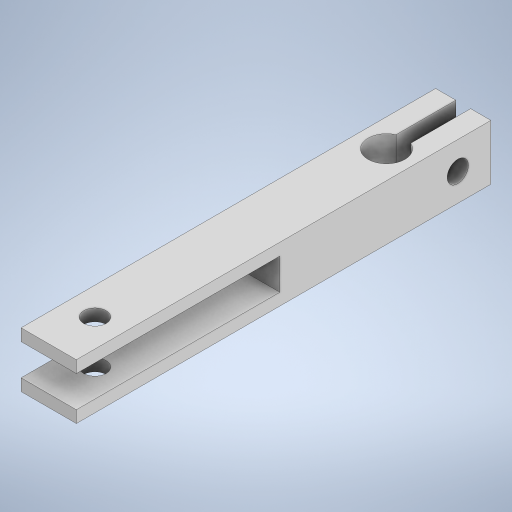
# Autodesk Inventor part: LInk1
Saved by Autodesk Inventor 2024 (Build 280153000, 153)
## iProperties
Created: 2023-12-17
Part Number: LInk1
Material: Generic
Document SubType Name: Modeling
Designer: pratikhya
Density: 1 g/cm^3
Appearance: Default
Author: pratikhya
Autodesk Inventor part; units mm, degrees
ref_plane "YZ Plane" through (0, 0, 0) normal (1, 0, 0) x (0, 1, 0)
ref_plane "XZ Plane" through (0, 0, 0) normal (0, 1, 0) x (-1, 0, 0)
ref_plane "XY Plane" through (0, 0, 0) normal (0, 0, 1) x (1, 0, 0)
sketch "Sketch1" plane through (0, 0, 0) normal (0, 1, 0) x (-1, 0, 0)
  point P0 (0, 0)
sketch "Sketch2" plane through (0, 0, 0) normal (0, 1, 0) x (-1, 0, 0)
  line L0 (2.7724, 24.8182) -> (-3.2276, 24.8182)
  line L1 (2.7724, 24.8182) -> (2.7724, -20.1818)
  line L2 (-3.2276, 24.8182) -> (-3.2276, -20.1818)
  line L3 (-3.2276, -20.1818) -> (-1.0276, -20.1818)
  line L4 (-1.0276, -20.1818) -> (-1.0276, -13.6818)
  line L5 (2.7724, -20.1818) -> (0.5724, -20.1818)
  line L6 (0.5724, -20.1818) -> (0.5724, -13.6818)
  arc A0 (0.5724, -13.6818) -> (-1.0276, -13.6818) centre (-0.2276, -11.8488) ccw
  point P0 (0, 0)
  dimension "d0" = 6
  dimension "d1" = 45
  dimension "d2" = 45
  dimension "d3" = 2.2
  dimension "d4" = 2.2
  dimension "d5" = 6.5
  dimension "d6" = 2
  constraints: 14 end point, 3 vertical, 2 horizontal, 2 perpendicular, 2 point on circle, 1 centre point
  measures "d0" distance of L0.start L0.end
  measures "d1" distance of L0.start L1.end
  measures "d2" distance of L0.end L2.end
  measures "d3" distance of L2.end L3.end
  measures "d4" distance of L1.end L5.end
  measures "d5" distance of L3.end L4.end
  measures "d6" radius of A0
extrude "Extrusion1" add sketch "Sketch2" along normal blind 6
sketch "Sketch4" plane through (0, 0, 0) normal (0, -1, 0) x (1, 0, 0)
  line L0 (-2.7724, 24.8182) -> (3.2276, 24.8182) projected
  circle A0 centre (0.2276, 19.8001) radius 1.2121
  point P0 (0, 0)
  constraints: 1 centre point
extrude "Extrusion3" cut sketch "Sketch4" against normal blind 10.9375
sketch "Sketch5" plane through (3.2276, 0, 24.8182) normal (1, 0, 0) x (0, 0, -1)
  circle A0 centre (41.4031, 3) radius 1.15
  line L0 (0, 0) -> (0, 6) projected
  line L1 (0, 4.7) -> (22.0881, 4.7)
  line L2 (22.0881, 4.7) -> (22.0881, 1.3)
  line L3 (22.0881, 1.3) -> (0, 1.3)
  line L4 (0, 4.7) -> (0, 1.3)
  point P0 (24.8182, 0)
  dimension "d13" = 2.3
  dimension "d18" = 3.4
  dimension "d19" = 1.3
  constraints: 8 end point, 2 perpendicular, 2 point on line, 1 centre point, 1 collinear, 1 horizontal
  measures "d13" diameter of A0
  measures "d18" distance of L1.end L2.end
  measures "d19" distance of L1.start L0.end
extrude "Extrusion4" cut sketch "Sketch5" against normal blind 14.6375 contours A0
extrude "Extrusion5" cut sketch "Sketch5" against normal blind 23.4625 contours L0 L1 L2 L3
body "Solid1"
